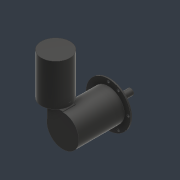
# Autodesk Inventor part: PN00113-6
Saved by Autodesk Inventor 2017 SP1 (Build 210196100, 196)
## iProperties
Created: 2018-04-10
Part Number: PN00113-6
Material: ABS Plastic
Document SubType Name: Modeling
Designer: Zach
Density: 1.06 g/cm^3
Appearance: Smooth - Black
Author: Zach
Autodesk Inventor part; units mm, degrees
ref_plane "YZ Plane" through (0, 0, 0) normal (1, 0, 0) x (0, 1, 0)
ref_plane "XZ Plane" through (0, 0, 0) normal (0, 1, 0) x (-1, 0, 0)
ref_plane "XY Plane" through (0, 0, 0) normal (0, 0, 1) x (1, 0, 0)
sketch "Sketch1" plane through (0, 0, 0) normal (0, 0, 1) x (1, 0, 0)
  circle A0 centre (0, 0) radius 34
  dimension "d0" = 68
  constraints: 1 centre point, 1 coincident
  measures "d0" diameter of A0
extrude "Extrusion1" add sketch "Sketch1" along normal blind 98.6
sketch "Sketch2" plane through (0, 0, 0) normal (0, 1, 0) x (-1, 0, 0)
  circle A0 centre (-37, -39.4) radius 38
  line L0 (34, 98.6) -> (-34, 98.6) projected
  point P0 (0, 0)
  dimension "d3" = 76
  dimension "d4" = 138
  dimension "d5" = 37
  constraints: 1 centre point
  measures "d3" diameter of A0
  measures "d4" distance from line of L0 A0.centre
  measures "d5" horizontal distance of A0.centre point (0, 0)
extrude "Extrusion2" add sketch "Sketch2" along normal blind 90.5 and the other way blind 20
sketch "Sketch3" plane through (37, 90.5, -39.4) normal (0, 1, 0) x (1, 0, 0)
  circle A0 centre (0, 0) radius 53
  circle A1 centre (0, 0) radius 38 projected
  point P0 (-37, -39.4)
  dimension "d10" = 106
  constraints: 1 centre point, 1 coincident
  measures "d10" diameter of A0
extrude "Extrusion3" add sketch "Sketch3" against normal blind 3
sketch "Sketch4" plane through (0, 0, 0) normal (0, 1, 0) x (-1, 0, 0)
  circle A0 centre (-37, -39.4) radius 38 projected
  line L0 (0, 0) -> (-37, 0)
  line L1 (-34, 0) -> (34, 0) projected
  line L2 (0, 0) -> (0, -39.4)
  line L3 (0, -39.4) -> (-37, -39.4)
  line L4 (-37, -39.4) -> (-37, 0)
  constraints: 8 end point, 1 collinear, 1 horizontal, 1 horizontal alignment, 1 perpendicular, 1 vertical, 1 vertical alignment
extrude "Extrusion4" add sketch "Sketch4" along normal blind 10 and the other way blind 20 contours L2 L3 L4 A0 | A0 L4 L0 L2 picked at (-12.3333, -36.5132)
sketch "Sketch5" plane through (37, 90.5, -39.4) normal (0, 1, 0) x (1, 0, 0)
  circle A0 centre (0, 0) radius 53 construction
  circle A1 centre (0, 0) radius 7.5
  point P0 (-37, -39.4)
  dimension "d17" = 15
  constraints: 1 centre point, 1 coincident
  measures "d17" diameter of A1
extrude "Extrusion5" add sketch "Sketch5" along normal blind 50
sketch "Sketch6" plane through (37, 90.5, -39.4) normal (0, 1, 0) x (1, 0, 0)
  circle A0 centre (0, 0) radius 53 construction
  circle A1 centre (23.5, 40.7032) radius 3.1
  line L0 (0, 0) -> (0, 53) construction
  line L1 (0, 0) -> (23.5, 40.7032) construction
  circle A2 centre (-47, 0) radius 3.1
  circle A3 centre (23.5, -40.7032) radius 3.1
  circle A4 centre (0, 47) radius 3.1
  circle A5 centre (-47, 0) radius 3.1
  circle A6 centre (0, -47) radius 3.1
  circle A7 centre (47, 0) radius 3.1
  point P0 (-37, -39.4)
  dimension "d20" = 6.2
  dimension "d21" = 47
  dimension "d22" = 30
  dimension "d25" = 360
  dimension "d27" = 6.2
  dimension "d28" = 47
  dimension "d31" = 360
  constraints: 7 centre point, 4 end point, 1 point on line, 1 vertical, 1 vertical alignment, 17 other
  measures "d20" diameter of A1
  measures "d21" distance of L0.start L1.end
  measures "d22" angle of L0 L1
  measures "d27" diameter of A4
  measures "d28" distance of L0.start A4.centre
extrude "Extrusion6" cut sketch "Sketch6" against normal through all
body "Solid1"
